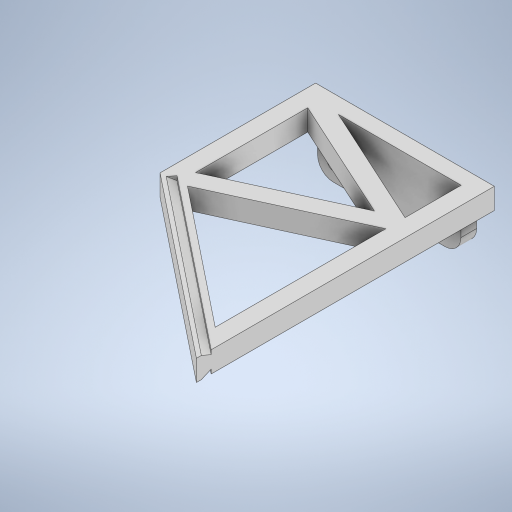
# Autodesk Inventor part: Base_ScreenHolder_R
Saved by Autodesk Inventor 2023 (Build 270158000, 158)
## iProperties
Created: 2025-02-14
Part Number: Base_ScreenHolder_R
Material: Generic
Document SubType Name: Modeling
Designer: Swoby
Density: 1 g/cm^3
Appearance: Default
Author: Swoby
Autodesk Inventor part; units mm, degrees
ref_plane "YZ Plane" through (0, 0, 0) normal (1, 0, 0) x (0, 1, 0)
ref_plane "XZ Plane" through (0, 0, 0) normal (0, 1, 0) x (-1, 0, 0)
ref_plane "XY Plane" through (0, 0, 0) normal (0, 0, 1) x (1, 0, 0)
sketch "Sketch1" plane through (0, 0, 0) normal (0, 0, 1) x (1, 0, 0)
  circle A0 centre (-16, 13) radius 1.75
  circle A1 centre (16, 13) radius 1.75
  line L0 (-16, 13) -> (16, 13) construction
  line L1 (0, 13) -> (0, 0) construction
  line L2 (0, 0) -> (-25.5715, 0)
  line L3 (-25.5715, 0) -> (-25.5715, 6)
  line L4 (-25.5715, 6) -> (-20.5, 6)
  line L5 (-20.5, 6) -> (-20.5, 13)
  line L6 (-16, 17.5) -> (0, 17.5)
  arc A2 (-16, 17.5) -> (-20.5, 13) centre (-16, 13) ccw
  circle A3 centre (16, 13) radius 1.75
  line L7 (0, 0) -> (25.5715, 0)
  line L8 (25.5715, 0) -> (25.5715, 6)
  line L9 (25.5715, 6) -> (20.5, 6)
  line L10 (20.5, 6) -> (20.5, 13)
  line L11 (16, 17.5) -> (0, 17.5)
  arc A4 (20.5, 13) -> (16, 17.5) centre (16, 13) ccw
  dimension "d0" = 3.5
  dimension "d1" = 3.5
  dimension "d2" = 32
  dimension "d3" = 13
  dimension "d4" = 25.5715
  dimension "d5" = 6
  dimension "d18" = 4.5
  constraints: 24 end point, 6 symmetric about line, 5 centre point, 4 perpendicular, 4 point on circle, 3 horizontal, 2 tangent, 1 concentric, 1 midpoint, 1 point on line, 2 other
  measures "d0" diameter of A0
  measures "d1" diameter of A1
  measures "d2" distance of L0.start L0.end
  measures "d3" distance of L1.start L1.end
  measures "d4" distance of L1.end L2.end
  measures "d5" distance of L2.end L3.end
  measures "d18" distance from line of A2.centre L6
extrude "Extrusion1" add sketch "Sketch1" along normal blind 4.5
sketch "Sketch2" plane through (-25.5715, 0, 0) normal (0, -1, 0) x (1, 0, 0)
  line L0 (0, 0) -> (51.143, 0) projected
  line L1 (51.143, 0) -> (51.143, 4.5) projected
  line L2 (0, 4.5) -> (51.143, 4.5) projected
  line L3 (0, 0) -> (0, 4.5) projected
  line L4 (0, 4.5) -> (0, 44.5)
  line L5 (0, 44.5) -> (51.143, 85.2393)
  line L6 (51.143, 85.2393) -> (51.143, 4.5)
  line L7 (46.143, 4.5) -> (46.143, 74.864)
  line L8 (46.143, 74.864) -> (5, 42.0904)
  line L9 (5, 42.0904) -> (5, 4.5)
  line L10 (5, 4.5) -> (46.143, 23.2952) construction
  line L11 (5, 42.0904) -> (46.143, 23.2952) construction
  line L12 (5, 23.2952) -> (46.143, 23.2952) construction
  line L13 (5, 4.5) -> (0, 4.5)
  line L14 (46.143, 4.5) -> (51.143, 4.5)
  line L15 (7.1928, 43.8372) -> (46.143, 26.0437)
  line L16 (5, 39.3419) -> (40.1265, 23.2952)
  line L17 (40.1265, 23.2952) -> (5, 7.2485)
  line L18 (46.143, 20.5467) -> (11.0165, 4.5)
  line L19 (5, 7.2485) -> (5, 4.5)
  point P0 (25.5715, 0)
  dimension "d9" = 128.54
  dimension "d10" = 40
  dimension "d11" = 5
  dimension "d14" = 2.5
  dimension "d15" = 2.5
  constraints: 32 end point, 10 point on line, 4 collinear, 4 parallel, 2 midpoint, 1 horizontal, 1 vertical, 2 other
  measures "d9" angle of L4 L5
  measures "d10" distance of L2.start L4.end
  measures "d11" distance between parallel lines of L6 L7
  measures "d14" distance between parallel lines of L11 L15
  measures "d15" distance between parallel lines of L16 L11
extrude "Extrusion2" add sketch "Sketch2" against normal blind 6 contours L4 L5 L6 L2 L7 L8 L9 | L9 L17 L16 L8 L15 L7 L18 L2
ref_plane "Work Plane1" through (25.5715, 0, 85.2393) normal (0.7821734, 0, 0.6230608) x (0, 1, 0)
sketch "Sketch4" plane through (25.5715, 0, 85.2393) normal (0.7821734, 0, 0.6230608) x (0, 1, 0)
  line L0 (0, -66.6719) -> (6, -66.6719) projected
  line L1 (6, -66.6719) -> (6, 0) projected
  line L2 (0, 0) -> (6, 0) projected
  line L3 (0, -66.6719) -> (0, 0) projected
  line L4 (0, -1.1) -> (1.2, -3.3)
  line L5 (1.2, -3.3) -> (0, -3.3)
  line L6 (3, 0) -> (3, -3.4483) construction
  point P0 (0, -50.7393)
  dimension "d29" = 1.1
  dimension "d30" = 3.3
  dimension "d31" = 3.6
  constraints: 6 end point, 2 point on line, 1 midpoint, 1 perpendicular, 1 vertical
  measures "d29" distance of L4.start L2.start
  measures "d30" distance from line of L5.end L2
  measures "d31" diameter of L4.end L6
extrude "Extrusion4" cut sketch "Sketch4" against normal blind 64 contours L3 L4 L5
ref_plane "Work Plane2" through (-25.5715, 3, 0) normal (0, -1, 0) x (1, 0, 0)
mirror "Mirror1" about plane through (-25.5715, 3, 0) normal (0, -1, 0) of "Extrusion4"
mirror "Mirror2" about plane through (0, 0, 0) normal (0, 1, 0) remove original yes
equation "\"d14\" = 0.5 * d11"
equation "\"d15\" = d14"
body "Solid1"
